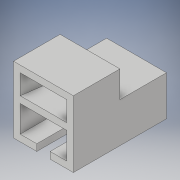
# Autodesk Inventor part: big usb cover
Saved by Autodesk Inventor 2018 (Build 220112000, 112)
## iProperties
Created: 2018-01-13
Part Number: big usb cover
Material: Generic
Document SubType Name: Modeling
Designer: cruz.anthony
Density: 1 g/cm^3
Appearance: Default
Author: cruz.anthony
Autodesk Inventor part; units mm, degrees
ref_plane "YZ Plane" through (0, 0, 0) normal (1, 0, 0) x (0, 1, 0)
ref_plane "XZ Plane" through (0, 0, 0) normal (0, 1, 0) x (-1, 0, 0)
ref_plane "XY Plane" through (0, 0, 0) normal (0, 0, 1) x (1, 0, 0)
sketch "Sketch1" plane through (0, 0, 0) normal (0, 1, 0) x (-1, 0, 0)
  line L0 (0, 0) -> (22.86, 0)
  line L1 (22.86, 0) -> (22.86, 35.56)
  line L2 (22.86, 35.56) -> (0, 35.56)
  line L3 (0, 35.56) -> (0, 0)
  dimension "d0" = 22.86
  dimension "d1" = 35.56
  constraints: 8 end point, 2 parallel, 1 horizontal, 1 perpendicular
  measures "d0" distance of L2.end L1.end
  measures "d1" distance of L1.end L0.end
extrude "Extrusion1" add sketch "Sketch1" along normal blind 15.24
sketch "Sketch2" plane through (-22.86, 0, 35.56) normal (0, 0, 1) x (1, 0, 0)
  line L0 (2.54, 2.54) -> (20.32, 2.54)
  line L1 (20.32, 2.54) -> (20.32, 12.7)
  line L2 (20.32, 12.7) -> (2.54, 12.7)
  line L3 (2.54, 12.7) -> (2.54, 2.54)
  point P0 (0, 0)
  dimension "d6" = 17.78
  dimension "d7" = 10.16
  constraints: 8 end point, 2 parallel, 1 horizontal, 1 perpendicular
  measures "d6" distance of L2.end L1.end
  measures "d7" distance of L1.end L0.end
extrude "Extrusion2" cut sketch "Sketch2" against normal blind 33.02
sketch "Sketch5" plane through (0, 15.24, 0) normal (0, 1, 0) x (1, 0, 0)
  line L0 (-22.86, -35.56) -> (0, -35.56) projected
  line L1 (0, -35.56) -> (0, 0) projected
  line L2 (-22.86, -35.56) -> (0, -35.56)
  line L3 (0, -35.56) -> (0, -17.78)
  line L4 (0, -17.78) -> (-22.86, -17.78)
  line L5 (-22.86, -17.78) -> (-22.86, -35.56)
  constraints: 8 end point, 2 parallel, 1 horizontal, 1 midpoint, 1 perpendicular
extrude "Extrusion5" add sketch "Sketch5" along normal blind 10.16
sketch "Sketch10" plane through (-22.86, 0, 35.56) normal (0, 0, 1) x (1, 0, 0)
  line L0 (2.54, 15.24) -> (20.32, 15.24)
  line L1 (20.32, 15.24) -> (20.32, 22.86)
  line L2 (20.32, 22.86) -> (2.54, 22.86)
  line L3 (2.54, 22.86) -> (2.54, 15.24)
  line L4 (2.54, 12.7) -> (20.32, 12.7) projected
  line L5 (22.86, 0) -> (22.86, 25.4) projected
  dimension "d27" = 17.78
  dimension "d28" = 7.62
  dimension "d29" = 2.54
  dimension "d30" = 2.54
  constraints: 8 end point, 2 parallel, 1 horizontal, 1 perpendicular
  measures "d27" distance of L0.start L0.end
  measures "d28" distance of L0.end L1.end
  measures "d29" distance between parallel lines of L4 L0
  measures "d30" distance between parallel lines of L5 L1
sketch "Sketch11" plane through (0, 15.24, 17.78) normal (0, 0, -1) x (-1, 0, 0)
  line L0 (17.78, 7.62) -> (5.08, 7.62)
  line L1 (5.08, 7.62) -> (5.08, 0)
  line L2 (5.08, 0) -> (17.78, 0)
  line L3 (17.78, 0) -> (17.78, 7.62)
  line L4 (0, 10.16) -> (22.86, 10.16) projected
  line L5 (22.86, 0) -> (22.86, 10.16) projected
  point P0 (0, -15.24)
  dimension "d31" = 2.54
  dimension "d33" = 5.08
  dimension "d35" = 12.7
  dimension "d36" = 7.62
  constraints: 8 end point, 2 parallel, 1 horizontal, 1 perpendicular
  measures "d31" distance between parallel lines of L4 L0
  measures "d33" distance between parallel lines of L5 L3
  measures "d35" distance of L0.start L0.end
  measures "d36" distance of L0.end L1.end
loft "Loft1" cut profiles "Sketch11", "Sketch10"
sketch "Sketch12" plane through (0, 0, 0) normal (0, 0, -1) x (-1, 0, 0)
  line L0 (22.86, 0) -> (0, 0) projected
  line L1 (0, 0) -> (11.43, 0)
  line L2 (11.43, 0) -> (11.43, 7.62)
  circle A0 centre (11.43, 7.62) radius 2.54
  dimension "d41" = 11.43
  dimension "d42" = 7.62
  dimension "d43" = 5.08
  constraints: 4 end point, 1 centre point, 1 coincident, 1 midpoint, 1 perpendicular
  measures "d41" distance of L0.end L1.end
  measures "d42" distance of L1.end L2.end
  measures "d43" diameter of A0
extrude "Extrusion8" cut sketch "Sketch12" against normal blind 25.4
sketch "Sketch13" plane through (0, 0, 0) normal (0, -1, 0) x (1, 0, 0)
  line L0 (0, 0) -> (-8.89, 0)
  line L1 (0, 0) -> (-22.86, 0) projected
  line L2 (-22.86, 0) -> (-13.97, 0)
  line L3 (-20.32, 35.56) -> (-2.54, 35.56) projected
  line L4 (-13.97, 0) -> (-8.89, 0)
  line L5 (-8.89, 0) -> (-8.89, 35.56)
  line L6 (-8.89, 35.56) -> (-13.97, 35.56)
  line L7 (-13.97, 35.56) -> (-13.97, 0)
  dimension "d46" = 8.89
  dimension "d47" = 8.89
  constraints: 12 end point, 3 point on line, 2 parallel, 1 horizontal, 1 perpendicular
  measures "d46" distance of L0.start L0.end
  measures "d47" distance of L1.end L2.end
extrude "Extrusion9" cut sketch "Sketch13" against normal blind 7.62
body "Solid1"
